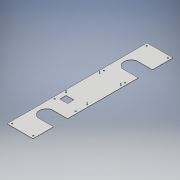
# Autodesk Inventor part: Cover_Right
Saved by Autodesk Inventor 2018 (Build 220112000, 112)
## iProperties
Created: 2017-12-05
Part Number: Cover_Right
Material: Generic
Document SubType Name: Modeling
Designer: P136265
Density: 1 g/cm^3
Appearance: Default
Author: P136265
Autodesk Inventor part; units mm, degrees
ref_plane "YZ Plane" through (0, 0, 0) normal (1, 0, 0) x (0, 1, 0)
ref_plane "XZ Plane" through (0, 0, 0) normal (0, 1, 0) x (-1, 0, 0)
ref_plane "XY Plane" through (0, 0, 0) normal (0, 0, 1) x (1, 0, 0)
sketch "Sketch1" plane through (0, 0, 0) normal (0, 0, 1) x (1, 0, 0)
  line L0 (-28.6, -15.9) -> (0, -15.9) construction
  line L1 (-28.6, 817.5) -> (-28.6, -17.5) construction
  line L2 (125, 817.5) -> (125, -17.5) construction
  line L3 (96.4, -15.9) -> (125, -15.9) construction
  line L4 (-28.6, 815.9) -> (0, 815.9) construction
  line L5 (96.4, 815.9) -> (125, 815.9) construction
  circle A0 centre (-14.3, 0) radius 2 construction
  circle A1 centre (110.7, 0) radius 2 construction
  circle A2 centre (-14.3, 252.5) radius 2 construction
  circle A3 centre (110.7, 252.5) radius 2 construction
  circle A4 centre (-14.3, 545.5) radius 2 construction
  circle A5 centre (110.7, 545.5) radius 2 construction
  circle A6 centre (-14.3, 800) radius 2 construction
  circle A7 centre (110.7, 800) radius 2 construction
  line L6 (-28.6, -15.9) -> (125, -15.9)
  line L7 (125, -15.9) -> (125, 815.9)
  line L8 (125, 815.9) -> (-28.6, 815.9)
  line L9 (-28.6, 815.9) -> (-28.6, -15.9)
  circle A8 centre (-14.3, 0) radius 4
  circle A9 centre (110.7, 0) radius 4
  circle A10 centre (-14.3, 252.5) radius 4
  circle A11 centre (110.7, 252.5) radius 4
  circle A12 centre (-14.3, 545.5) radius 4
  circle A13 centre (110.7, 545.5) radius 4
  circle A14 centre (-14.3, 800) radius 4
  circle A15 centre (110.7, 800) radius 4
  point P0 (0, 0)
  dimension "d0" = 2
  dimension "d1" = 2
  dimension "d2" = 2
  dimension "d3" = 2
  dimension "d4" = 2
  dimension "d5" = 2
  dimension "d6" = 2
  dimension "d7" = 2
  constraints: 8 centre point, 8 end point, 2 parallel, 1 horizontal, 1 perpendicular
  measures "d0" radial gap between concentric circles of A0 A8
  measures "d1" radial gap between concentric circles of A1 A9
  measures "d2" radial gap between concentric circles of A2 A10
  measures "d3" radial gap between concentric circles of A3 A11
  measures "d4" radial gap between concentric circles of A4 A12
  measures "d5" radial gap between concentric circles of A5 A13
  measures "d6" radial gap between concentric circles of A6 A14
  measures "d7" radial gap between concentric circles of A7 A15
extrude "Extrusion1" add sketch "Sketch1" along normal blind 2
sketch "Sketch2" plane through (0, 0, 2) normal (0, 0, 1) x (1, 0, 0)
  arc A0 (81.2, 144.25) -> (81.2, 152.25) centre (81.2, 148.25) ccw construction
  arc A1 (79.0077, 648.4043) -> (79.0077, 655.0957) centre (81.2, 651.75) ccw construction
  arc A2 (33.1012, 180.4907) -> (33.1012, 116.0093) centre (42.2, 148.25) ccw construction
  arc A3 (33.1012, 683.9907) -> (33.1012, 619.5093) centre (42.2, 651.75) ccw construction
  arc A4 (30.3852, 190.1148) -> (30.3852, 106.3852) centre (42.2, 148.25) ccw
  arc A5 (30.3852, 693.6148) -> (30.3852, 609.8852) centre (42.2, 651.75) ccw
  line L0 (125, -15.9) -> (125, 815.9) construction
  line L1 (30.3852, 106.3852) -> (125, 106.3852)
  line L2 (30.3852, 190.1148) -> (125, 190.1148)
  line L3 (30.3852, 609.8852) -> (125, 609.8852)
  line L4 (30.3852, 693.6148) -> (125, 693.6148)
  line L5 (125, 106.3852) -> (125, 190.1148)
  line L6 (125, 609.8852) -> (125, 693.6148)
  point P0 (0, 0)
  dimension "d10" = 10
  dimension "d11" = 10
  dimension "d16" = 83.7296
  dimension "d17" = 83.7296
  dimension "d18" = 41.8648
  dimension "d19" = 41.8648
  constraints: 12 end point, 4 perpendicular, 4 point on circle, 4 point on line, 2 centre point, 1 collinear, 1 vertical
  measures "d10" radial gap between concentric circles of A2 A4
  measures "d11" radial gap between concentric circles of A3 A5
  measures "d16" distance between parallel lines of L4 L3
  measures "d17" distance between parallel lines of L2 L1
  measures "d18" distance from line of L1 A2.centre
  measures "d19" distance from line of L3 A3.centre
extrude "Extrusion2" cut sketch "Sketch2" against normal blind 2
fillet "Fillet1" radius 2 8 edges at (-28.6, -15.9, 1) (125, -15.9, 1) (-28.6, 815.9, 1) (125, 815.9, 1) (125, 693.6148, 1) (125, 609.8852, 1) (125, 106.3852, 1) (125, 190.1148, 1)
sketch "Sketch3" plane through (0, 0, 2) normal (0, 0, 1) x (1, 0, 0)
  arc A0 (123, 190.1148) -> (125, 192.1148) centre (123, 192.1148) ccw construction
  line L0 (125, 192.1148) -> (125, 607.8852) construction
  arc A1 (125, 607.8852) -> (123, 609.8852) centre (123, 607.8852) ccw construction
  line L1 (123, 609.8852) -> (30.3852, 609.8852) construction
  arc A2 (30.3852, 693.6148) -> (30.3852, 609.8852) centre (42.2, 651.75) ccw construction
  line L2 (30.3852, 693.6148) -> (123, 693.6148) construction
  arc A3 (123, 693.6148) -> (125, 695.6148) centre (123, 695.6148) ccw construction
  line L3 (125, 695.6148) -> (125, 813.9) construction
  arc A4 (125, 813.9) -> (123, 815.9) centre (123, 813.9) ccw construction
  line L4 (123, 815.9) -> (-26.6, 815.9) construction
  arc A5 (-26.6, 815.9) -> (-28.6, 813.9) centre (-26.6, 813.9) ccw construction
  line L5 (-28.6, 813.9) -> (-28.6, -13.9) construction
  arc A6 (-28.6, -13.9) -> (-26.6, -15.9) centre (-26.6, -13.9) ccw construction
  line L6 (-26.6, -15.9) -> (123, -15.9) construction
  arc A7 (123, -15.9) -> (125, -13.9) centre (123, -13.9) ccw construction
  line L7 (125, -13.9) -> (125, 104.3852) construction
  arc A8 (125, 104.3852) -> (123, 106.3852) centre (123, 104.3852) ccw construction
  line L8 (123, 106.3852) -> (30.3852, 106.3852) construction
  arc A9 (30.3852, 190.1148) -> (30.3852, 106.3852) centre (42.2, 148.25) ccw construction
  line L9 (30.3852, 190.1148) -> (123, 190.1148) construction
  circle A10 centre (110.7, 800) radius 4 construction
  circle A11 centre (-14.3, 800) radius 4 construction
  circle A12 centre (110.7, 545.5) radius 4 construction
  circle A13 centre (-14.3, 545.5) radius 4 construction
  circle A14 centre (110.7, 252.5) radius 4 construction
  circle A15 centre (-14.3, 252.5) radius 4 construction
  circle A16 centre (110.7, 0) radius 4 construction
  circle A17 centre (-14.3, 0) radius 4 construction
  line L10 (-28.6, 813.9) -> (-28.6, -13.9) construction
  line L11 (-28.6, 400) -> (125, 400) construction
  line L12 (-28.6, 520) -> (125, 520) construction
  circle A18 centre (-14.3, 545.5) radius 4 construction
  line L13 (-28.6, 320) -> (125, 320) construction
  line L14 (-14.3, 545.5) -> (-14.3, 320) construction
  line L15 (110.7, 545.5) -> (110.7, 320) construction
  circle A19 centre (-14.3, 520) radius 2
  circle A20 centre (-14.3, 320) radius 2
  circle A21 centre (110.7, 320) radius 2
  circle A22 centre (110.7, 520) radius 2
  point P0 (0, 0)
  dimension "d24" = 120
  dimension "d25" = 200
  dimension "d26" = 4
  dimension "d27" = 4
  dimension "d28" = 4
  dimension "d29" = 4
  constraints: 10 end point, 6 point on line, 4 centre point, 2 coincident, 2 midpoint, 2 parallel, 2 perpendicular
  measures "d24" distance between parallel lines of L11 L12
  measures "d25" distance between parallel lines of L12 L13
  measures "d26" diameter of A19
  measures "d27" diameter of A20
  measures "d28" diameter of A21
  measures "d29" diameter of A22
extrude "Extrusion3" add sketch "Sketch3" along normal blind 10
chamfer "Chamfer1" distance 1 angle 45 4 edges at (-16.3, 320, 2) (-16.3, 520, 2) (108.7, 520, 2) (108.7, 320, 2)
thread "Thread1" size "M4x0.7" class "6g" standard "ANSI Metric M Profile" full length
thread "Thread2" size "M4x0.7" class "6g" standard "ANSI Metric M Profile" full length
thread "Thread3" size "M4x0.7" class "6g" standard "ANSI Metric M Profile" full length
thread "Thread4" size "M4x0.7" class "6g" standard "ANSI Metric M Profile" full length
sketch "Sketch4" plane through (0, 0, 2) normal (0, 0, 1) x (1, 0, 0)
  circle A0 centre (110.7, 520) radius 3 construction
  circle A1 centre (-14.3, 320) radius 3 construction
  arc A2 (123, 190.1148) -> (125, 192.1148) centre (123, 192.1148) ccw construction
  line L0 (125, 192.1148) -> (125, 607.8852) construction
  arc A3 (125, 607.8852) -> (123, 609.8852) centre (123, 607.8852) ccw construction
  line L1 (123, 609.8852) -> (30.3852, 609.8852) construction
  arc A4 (30.3852, 693.6148) -> (30.3852, 609.8852) centre (42.2, 651.75) ccw construction
  line L2 (30.3852, 693.6148) -> (123, 693.6148) construction
  arc A5 (123, 693.6148) -> (125, 695.6148) centre (123, 695.6148) ccw construction
  line L3 (125, 695.6148) -> (125, 813.9) construction
  arc A6 (125, 813.9) -> (123, 815.9) centre (123, 813.9) ccw construction
  line L4 (123, 815.9) -> (-26.6, 815.9) construction
  arc A7 (-26.6, 815.9) -> (-28.6, 813.9) centre (-26.6, 813.9) ccw construction
  line L5 (-28.6, 813.9) -> (-28.6, -13.9) construction
  arc A8 (-28.6, -13.9) -> (-26.6, -15.9) centre (-26.6, -13.9) ccw construction
  line L6 (-26.6, -15.9) -> (123, -15.9) construction
  arc A9 (123, -15.9) -> (125, -13.9) centre (123, -13.9) ccw construction
  line L7 (125, -13.9) -> (125, 104.3852) construction
  arc A10 (125, 104.3852) -> (123, 106.3852) centre (123, 104.3852) ccw construction
  line L8 (123, 106.3852) -> (30.3852, 106.3852) construction
  arc A11 (30.3852, 190.1148) -> (30.3852, 106.3852) centre (42.2, 148.25) ccw construction
  line L9 (30.3852, 190.1148) -> (123, 190.1148) construction
  circle A12 centre (110.7, 800) radius 4 construction
  circle A13 centre (-14.3, 800) radius 4 construction
  circle A14 centre (110.7, 545.5) radius 4 construction
  circle A15 centre (-14.3, 545.5) radius 4 construction
  circle A16 centre (110.7, 252.5) radius 4 construction
  circle A17 centre (-14.3, 252.5) radius 4 construction
  circle A18 centre (110.7, 0) radius 4 construction
  circle A19 centre (-14.3, 0) radius 4 construction
  circle A20 centre (-14.3, 520) radius 3 construction
  circle A21 centre (110.7, 320) radius 3 construction
  circle A22 centre (-14.3, 320) radius 2 construction
  circle A23 centre (110.7, 252.5) radius 4 construction
  line L10 (110.7, 252.5) -> (-14.3, 252.5) construction
  line L11 (-14.3, 252.5) -> (-14.3, 320) construction
  line L12 (-14.3, 320) -> (110.7, 320) construction
  line L13 (110.7, 320) -> (110.7, 252.5) construction
  line L14 (48.2, 252.5) -> (48.2, 320) construction
  line L15 (0.7, 267.5) -> (95.7, 267.5) construction
  line L16 (95.7, 267.5) -> (95.7, 305) construction
  line L17 (95.7, 305) -> (0.7, 305) construction
  line L18 (0.7, 305) -> (0.7, 267.5) construction
  line L19 (2.7, 267.5) -> (46.2, 267.5)
  line L20 (48.2, 269.5) -> (48.2, 303)
  line L21 (46.2, 305) -> (2.7, 305)
  line L22 (0.7, 303) -> (0.7, 269.5)
  arc A24 (0.7, 269.5) -> (2.7, 267.5) centre (2.7, 269.5) ccw
  arc A25 (2.7, 305) -> (0.7, 303) centre (2.7, 303) ccw
  arc A26 (46.2, 267.5) -> (48.2, 269.5) centre (46.2, 269.5) ccw
  arc A27 (48.2, 303) -> (46.2, 305) centre (46.2, 303) ccw
  point P0 (0, 0)
  point P1 (48.2, 305)
  dimension "d43" = 15
  dimension "d44" = 2
  dimension "d45" = 2
  dimension "d46" = 2
  dimension "d47" = 2
  constraints: 26 end point, 8 point on circle, 8 tangent, 6 parallel, 4 centre point, 4 point on line, 3 midpoint, 3 perpendicular, 2 horizontal, 3 other
  measures "d43" distance between parallel lines of L10 L15
  measures "d44" radius of A24
  measures "d45" radius of A25
  measures "d46" radius of A26
  measures "d47" radius of A27
extrude "Extrusion4" cut sketch "Sketch4" against normal up to next
body "Solid1"
